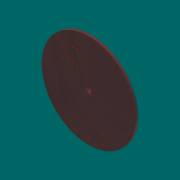
# Autodesk Inventor part: 知能ロボコンターンテーブル
Saved by Autodesk Inventor 2013 (Build 170138000, 138)
## iProperties
Created: 2014-05-11
Part Number: 知能ロボコンターンテーブル
Material: アセタール樹脂、白
Document SubType Name: Modeling
Designer: horumo136
Density: 1 g/cm^3
Author: horumo136
Autodesk Inventor part; units mm, degrees
ref_plane "YZ Plane" through (0, 0, 0) normal (1, 0, 0) x (0, 1, 0)
ref_plane "XZ Plane" through (0, 0, 0) normal (0, 1, 0) x (-1, 0, 0)
ref_plane "XY Plane" through (0, 0, 0) normal (0, 0, 1) x (1, 0, 0)
sketch "スケッチ1" plane through (0, 0, 0) normal (0, 1, 0) x (-1, 0, 0)
  circle A0 centre (0, 0) radius 100
  dimension "d0" = 200
  constraints: 1 centre point, 1 coincident
  measures "d0" diameter of A0
extrude "押し出し1" add sketch "スケッチ1" along normal blind 5
sketch "スケッチ12" plane through (0, 5, 0) normal (0, 1, 0) x (1, 0, 0)
  circle A0 centre (0, 0) radius 100 projected
  circle A1 centre (0, 0) radius 3.5
  circle A2 centre (0, 0) radius 5
  circle A3 centre (0, 0) radius 7
  circle A4 centre (0, 7) radius 1
  circle A5 centre (-4.9497, 4.9497) radius 1
  circle A6 centre (-7, 0) radius 1
  circle A7 centre (-4.9497, -4.9497) radius 1
  circle A8 centre (0, -7) radius 1
  circle A9 centre (4.9497, -4.9497) radius 1
  circle A10 centre (7, 0) radius 1
  circle A11 centre (4.9497, 4.9497) radius 1
  dimension "d94" = 14
  dimension "d92" = 7
  dimension "d93" = 10
  dimension "d95" = 2
  dimension "d98" = 360
  constraints: 10 centre point, 3 coincident, 1 vertical alignment, 19 other
  measures "d92" diameter of A1
  measures "d93" diameter of A2
  measures "d95" diameter of A4
hole "穴5" at (-7, 5, 0) at (-4.9497, 5, 4.9497) at (0, 5, 7) at (0, 5, -7) at (4.9497, 5, -4.9497) at (7, 5, 0) at (4.9497, 5, 4.9497) at (-4.9497, 5, -4.9497) direction (0, -1, 0) diameter 2 depth 8 tip angle 118
sketch "スケッチ13" plane through (0, 5, 0) normal (0, 1, 0) x (1, 0, 0)
  circle A0 centre (0, 0) radius 100 projected
  circle A1 centre (0, 0) radius 5
  dimension "d107" = 10
  constraints: 1 centre point, 1 coincident
  measures "d107" diameter of A1
extrude "押し出し4" cut sketch "スケッチ13" against normal blind 10 contours A1
sketch "スケッチ14" plane through (0, 5, 0) normal (0, 1, 0) x (1, 0, 0)
  circle A0 centre (0, 0) radius 100 projected
  line L0 (0, 0) -> (0, 55)
  line L1 (0, 55) -> (0, 65)
  line L2 (0, 65) -> (0, 85)
  line L3 (0, 65) -> (30, 65)
  line L4 (0, 65) -> (-30, 65)
  line L5 (-30, 65) -> (30, 65)
  line L6 (30, 65) -> (30, 85)
  line L7 (30, 85) -> (-30, 85)
  line L8 (-30, 85) -> (-30, 65)
  line L9 (0, 0) -> (0, -49.1)
  line L10 (0, -49.1) -> (-14.5, -49.1)
  line L11 (-14.5, -49.1) -> (-14.5, -34.1)
  line L12 (-14.5, -34.1) -> (-24.5, -34.1)
  line L13 (-24.5, -34.1) -> (-34.5, -34.1)
  line L14 (-34.5, -34.1) -> (-44.5, -34.1)
  line L15 (-44.5, -34.1) -> (-54.5, -34.1)
  line L16 (-54.5, -34.1) -> (-64.5, -34.1)
  line L17 (-24.5, -64.1) -> (-34.5, -64.1)
  line L18 (-34.5, -64.1) -> (-44.5, -64.1)
  line L19 (-44.5, -64.1) -> (-54.5, -64.1)
  line L20 (-54.5, -64.1) -> (-64.5, -64.1)
  point P0 (-14.5, -64.1)
  point P1 (-7.25, -49.1)
  dimension "d110" = 55
  dimension "d111" = 10
  dimension "d112" = 20
  dimension "d114" = 30
  dimension "d115" = 30
  dimension "d116" = 49.1
  dimension "d117" = 14.5
  dimension "d118" = 15
  dimension "d119" = 10
  dimension "d120" = 10
  dimension "d121" = 10
  dimension "d122" = 10
  dimension "d123" = 10
  constraints: 42 end point, 21 coincident, 11 symmetric about line, 8 parallel, 4 perpendicular, 3 collinear, 1 horizontal, 1 midpoint, 1 vertical
  measures "d110" distance of L0.start L0.end
  measures "d111" distance of L0.end L1.end
  measures "d112" distance of L1.end L2.end
  measures "d114" distance of L1.end L3.end
  measures "d115" distance of L1.end L4.end
  measures "d116" distance of L0.start L9.end
  measures "d117" distance of L9.end L10.end
  measures "d118" distance of L10.end L11.end
  measures "d119" distance of L11.end L12.end
  measures "d120" distance of L12.end L13.end
  measures "d121" distance of L13.end L14.end
  measures "d122" distance of L14.end L15.end
  measures "d123" distance of L15.end L16.end
hole "穴6" at (-30, 5, -85) at (-30, 5, -65) at (0, 5, -85) at (0, 5, -65) at (30, 5, -65) at (30, 5, -85) at (-64.5, 5, 34.1) at (-54.5, 5, 34.1) at (-44.5, 5, 34.1) at (-34.5, 5, 34.1) at (-24.5, 5, 34.1) at (-14.5, 5, 34.1) at (-64.5, 5, 64.1) at (-54.5, 5, 64.1) at (-44.5, 5, 64.1) at (-34.5, 5, 64.1) at (-24.5, 5, 64.1) at (-14.5, 5, 64.1) at (-30, 5, -85) at (-30, 5, -65) direction (0, -1, 0) diameter 3 depth 8 tip angle 118
